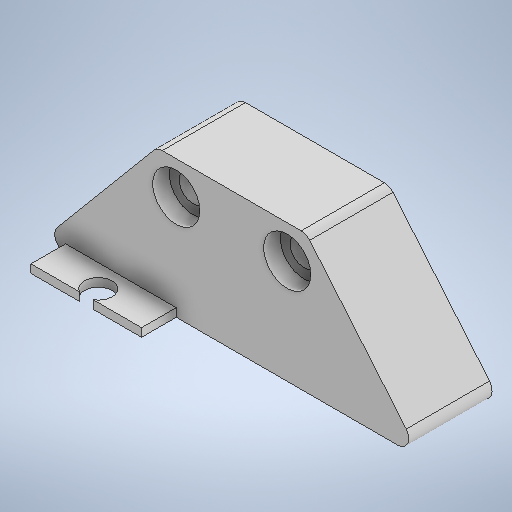
# Autodesk Inventor part: EngineMount
Saved by Autodesk Inventor 2026.1 (Build 301233020, 233B)
## iProperties
Created: 2025-10-14
Part Number: EngineMount
Material: Generic
Document SubType Name: Modeling
Designer: yo
Density: 1 g/cm^3
Appearance: Default
Author: yo
Autodesk Inventor part; units mm, degrees
ref_plane "YZ Plane" through (0, 0, 0) normal (1, 0, 0) x (0, 1, 0)
ref_plane "XZ Plane" through (0, 0, 0) normal (0, 1, 0) x (-1, 0, 0)
ref_plane "XY Plane" through (0, 0, 0) normal (0, 0, 1) x (1, 0, 0)
sketch "Sketch1" plane through (0, 0, 0) normal (0, 0, 1) x (1, 0, 0)
  line L0 (-59.8585, 0) -> (59.8585, 0)
  line L1 (-25.0359, 49.5) -> (25.0359, 49.5)
  circle A0 centre (-20, 37.5) radius 8.5
  line L2 (0, 49.5) -> (0, 0) construction
  circle A1 centre (-20, 37.5) radius 5
  circle A2 centre (20, 37.5) radius 8.5
  circle A3 centre (20, 37.5) radius 5
  arc A4 (-62.9227, 6.5712) -> (-59.8585, 0) centre (-59.8585, 4) ccw
  arc A5 (-25.0359, 49.5) -> (-28.1, 48.0712) centre (-25.0359, 45.5) ccw
  line L3 (-62.9227, 6.5712) -> (-28.1, 48.0712)
  arc A6 (59.8585, 0) -> (62.9227, 6.5712) centre (59.8585, 4) ccw
  arc A7 (28.1, 48.0712) -> (25.0359, 49.5) centre (25.0359, 45.5) ccw
  line L4 (62.9227, 6.5712) -> (28.1, 48.0712)
  line L5 (-59.8585, 3) -> (-20, 3)
  line L6 (-20, 3) -> (-20, 0)
  line L7 (-20, 0) -> (-59.8585, 0)
  line L8 (-59.8585, 0) -> (-59.8585, 3)
  point P0 (-59.8585, 1.5)
  point P1 (-39.9293, 0)
  point P2 (-20, 0)
  point P3 (-20, 1.5)
  dimension "d1" = 17
  dimension "d3" = 3.5
  dimension "d7" = 10
  dimension "d8" = 40
  dimension "d10" = 4
  dimension "d11" = 13
  dimension "d12" = 50
  dimension "d17" = 3
  dimension "d22" = 34.5
  constraints: 18 end point, 8 centre point, 8 point on circle, 6 symmetric about line, 5 midpoint, 4 coincident, 4 tangent, 3 horizontal, 2 parallel, 2 vertical alignment, 1 equal radius, 1 horizontal alignment, 1 perpendicular, 1 vertical, 4 other
  measures "d1" diameter of A0
  measures "d3" distance edge to line of A0 L1
  measures "d7" diameter of A1
  measures "d8" distance of A2.centre A0.centre
  measures "d10" radius of A4
  measures "d11" distance from line of A0.centre L3
  measures "d12" angle of L0 L3
  measures "d17" distance of L5.end L6.end
  measures "d22" distance from line of A0.centre L5
extrude "Extrusion1" add sketch "Sketch1" along normal mid plane 30 contours L8 L5 L6 L0 | A4 L3 A5 L1 A7 L4 A6 L0 L6 L5 L8
extrude "Extrusion2" add sketch "Sketch1" along normal mid plane 18 contours A0 | A2
extrude "Extrusion3" add sketch "Sketch1" along normal blind 27.5 contours L8 L5 L6 L0
sketch "Sketch2" plane through (-59.8585, 3, 15) normal (0, 1, 0) x (1, 0, 0)
  line L0 (0, -12.5) -> (39.8585, -12.5) projected
  arc A0 (22.4293, -12.5) -> (17.4293, -12.5) centre (19.9293, -8.1699) ccw
  line L1 (39.8585, 0) -> (119.717, 0) construction
  line L2 (39.8585, 0) -> (39.8585, -12.5) construction
  point P0 (59.8585, 15)
  point P1 (19.9293, -12.5)
  point P2 (19.9293, -3.1699)
  dimension "d21" = 5
  dimension "d25" = 5
  constraints: 3 point on circle, 2 point on line, 1 centre point, 1 midpoint, 1 vertical alignment
  measures "d21" radius of A0
  measures "d25" distance of A0.end A0.start
extrude "Extrusion4" cut sketch "Sketch2" against normal through all
body "Solid1"
